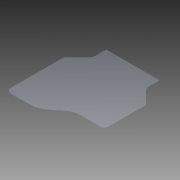
# Autodesk Inventor part: porta frontal
Saved by Autodesk Inventor 2012 SP1 (Build 160190100, 190)
## iProperties
Created: 2015-03-29
Part Number: porta frontal
Material: Default
Document SubType Name: Modeling
Designer: sheina
Density: 1 g/cm^3
Author: sheina
Autodesk Inventor part; units mm, degrees
ref_plane "YZ Plane" through (0, 0, 0) normal (1, 0, 0) x (0, 1, 0)
ref_plane "XZ Plane" through (0, 0, 0) normal (0, 1, 0) x (-1, 0, 0)
ref_plane "XY Plane" through (0, 0, 0) normal (0, 0, 1) x (1, 0, 0)
sketch "Boceto1" plane through (0, 0, 0) normal (0, 0, 1) x (1, 0, 0)
  line L0 (112.2616, 170.6474) -> (112.2616, 129.3648)
  arc A0 (112.2616, 129.3648) -> (118.4288, 114.4759) centre (133.3177, 129.3648) ccw
  line L1 (118.4288, 114.4759) -> (162.1204, 70.7843)
  arc A1 (166.2045, 60.9244) -> (162.1204, 70.7843) centre (152.2606, 60.9244) ccw
  line L2 (166.2045, 60.9244) -> (166.2045, -74.0436)
  arc A2 (152.2606, -87.9875) -> (166.2045, -74.0436) centre (152.2606, -74.0436) ccw
  line L3 (152.2606, -87.9875) -> (77.1714, -87.9875)
  arc A3 (77.1714, -87.9875) -> (28.3364, -107.4286) centre (77.1714, -159.0436) ccw
  arc A4 (-0.1519, -130.4951) -> (28.3364, -107.4286) centre (-135.1799, 65.3964) ccw
  arc A5 (-56.306, -147.9736) -> (-0.1519, -130.4951) centre (-56.306, -49.0297) ccw
  line L4 (-56.306, -147.9736) -> (-120.6823, -147.9736)
  arc A6 (-139.6262, -129.0297) -> (-120.6823, -147.9736) centre (-120.6823, -129.0297) ccw
  line L5 (-139.6262, -129.0297) -> (-139.6262, 60.9244)
  arc A7 (-135.5422, 70.7843) -> (-139.6262, 60.9244) centre (-125.6823, 60.9244) ccw
  line L6 (-135.5422, 70.7843) -> (-91.7934, 114.533)
  arc A8 (-91.7934, 114.533) -> (-85.6262, 129.4219) centre (-106.6823, 129.4219) ccw
  line L7 (-85.6262, 129.4219) -> (-85.6262, 170.6474)
  line L8 (-85.6262, 170.6474) -> (112.2616, 170.6474)
  constraints: 18 end point, 18 point on circle, 9 centre point
extrude "Extrusión1" add sketch "Boceto1" along normal blind 2
fillet "Empalme1" radius 2 2 edges at (-85.6262, 170.6474, 1) (112.2616, 170.6474, 1)
sketch "Boceto2" plane through (0, 0, 2) normal (0, 0, 1) x (1, 0, 0)
  line L0 (-139.6262, -129.0297) -> (-139.6262, 60.9244) projected
  circle A0 centre (-124.6262, 30.7843) radius 1.25
  circle A1 centre (-124.6262, 15.7843) radius 1.25
  circle A2 centre (-124.6262, -92.9736) radius 1.25
  circle A3 centre (-124.6262, -107.9736) radius 1.25
  point P0 (-135.5422, 70.7843)
  point P1 (-120.6823, -147.9736)
  point P2 (0, 0)
  dimension "d3" = 2.5
  dimension "d4" = 2.5
  dimension "d5" = 2.5
  dimension "d6" = 2.5
  dimension "d7" = 15
  dimension "d8" = 15
  dimension "d10" = 40
  dimension "d11" = 15
  dimension "d12" = 15
  dimension "d13" = 40
  constraints: 4 centre point
  measures "d3" diameter of A1
  measures "d4" diameter of A2
  measures "d5" diameter of A3
  measures "d6" diameter of A0
  measures "d7" distance of A0.centre A1.centre
  measures "d8" distance of A2.centre A3.centre
  measures "d10" vertical distance of A0.centre point (-135.542, 70.784)
  measures "d11" distance from line of L0 A0.centre
  measures "d12" distance from line of L0 A3.centre
  measures "d13" vertical distance of point (-120.682, -147.974) A3.centre
extrude "Extrusión2" cut sketch "Boceto2" against normal blind 2
sketch "Boceto3" plane through (0, 0, 0) normal (0, 0, -1) x (-1, 0, 0)
  line L0 (-166.2045, 60.9244) -> (-166.2045, -74.0436) projected
  line L1 (-152.2606, -87.9875) -> (-77.1714, -87.9875) projected
  circle A0 centre (-151.2045, 32.0125) radius 1.75
  circle A1 centre (-151.2045, -37.9875) radius 1.25
  point P0 (0, 0)
  dimension "d16" = 3.5
  dimension "d17" = 2.5
  dimension "d18" = 70
  dimension "d19" = 50
  dimension "d20" = 15
  constraints: 2 centre point
  measures "d16" diameter of A0
  measures "d17" diameter of A1
  measures "d18" distance of A1.centre A0.centre
  measures "d19" distance from line of A1.centre L1
  measures "d20" distance from line of A1.centre L0
extrude "Extrusión3" cut sketch "Boceto3" against normal blind 2
